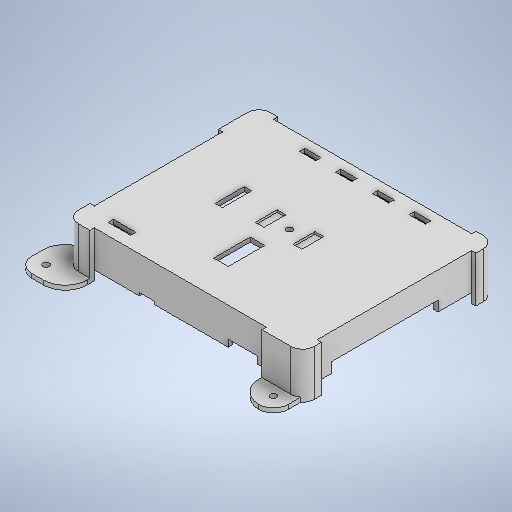
# Autodesk Inventor part: TopCase
Saved by Autodesk Inventor 2025.2 (Build 292293000, 293)
## iProperties
Created: 2026-05-08
Part Number: TopCase
Material: Generic
Document SubType Name: Modeling
Designer: Simon
Density: 1 g/cm^3
Appearance: Default
Author: Simon
Autodesk Inventor part; units mm, degrees
ref_plane "YZ Plane" through (0, 0, 0) normal (1, 0, 0) x (0, 1, 0)
ref_plane "XZ Plane" through (0, 0, 0) normal (0, 1, 0) x (-1, 0, 0)
ref_plane "XY Plane" through (0, 0, 0) normal (0, 0, 1) x (1, 0, 0)
sketch "Sketch1" plane through (0, 0, 0) normal (0, 1, 0) x (-1, 0, 0)
  line L0 (0, 0) -> (-156, 0)
  line L1 (-156, 0) -> (-156, -126)
  line L2 (-156, -126) -> (0, -126)
  line L3 (0, -126) -> (0, 0)
  line L4 (0, 0) -> (-3, 0)
  line L5 (-3, 0) -> (-3, -3)
  line L6 (-3, -3) -> (0, -3)
  line L7 (0, -3) -> (0, 0)
  line L8 (-156, 0) -> (-153, 0)
  line L9 (-153, 0) -> (-153, -3)
  line L10 (-153, -3) -> (-156, -3)
  line L11 (-156, -3) -> (-156, 0)
  line L12 (-156, -126) -> (-153, -126)
  line L13 (-153, -126) -> (-153, -123)
  line L14 (-153, -123) -> (-156, -123)
  line L15 (-156, -123) -> (-156, -126)
  line L16 (0, -126) -> (-3, -126)
  line L17 (-3, -126) -> (-3, -123)
  line L18 (-3, -123) -> (0, -123)
  line L19 (0, -123) -> (0, -126)
  line L20 (-156, 0) -> (-153.2, 0)
  line L21 (-153.2, 0) -> (-153.2, -126)
  line L22 (-153.2, -126) -> (-156, -126)
  line L23 (-156, -126) -> (-156, 0)
  line L24 (0, 0) -> (-2.8, 0)
  line L25 (-2.8, 0) -> (-2.8, -126)
  line L26 (-2.8, -126) -> (0, -126)
  line L27 (0, -126) -> (0, 0)
  line L28 (0, -126) -> (-156, -126)
  line L29 (-156, -126) -> (-156, -123.2)
  line L30 (-156, -123.2) -> (0, -123.2)
  line L31 (0, -123.2) -> (0, -126)
  line L32 (0, 0) -> (-156, 0)
  line L33 (-156, 0) -> (-156, -2.8)
  line L34 (-156, -2.8) -> (0, -2.8)
  line L35 (0, -2.8) -> (0, 0)
  line L36 (-3, -3) -> (-9, -3)
  line L37 (-9, -3) -> (-9, -9)
  line L38 (-9, -9) -> (-3, -9)
  line L39 (-3, -9) -> (-3, -3)
  line L40 (-153, -3) -> (-147, -3)
  line L41 (-147, -3) -> (-147, -9)
  line L42 (-147, -9) -> (-153, -9)
  line L43 (-153, -9) -> (-153, -3)
  line L44 (-153, -123) -> (-147, -123)
  line L45 (-147, -123) -> (-147, -117)
  line L46 (-147, -117) -> (-153, -117)
  line L47 (-153, -117) -> (-153, -123)
  line L48 (-3, -123) -> (-9, -123)
  line L49 (-9, -123) -> (-9, -117)
  line L50 (-9, -117) -> (-3, -117)
  line L51 (-3, -117) -> (-3, -123)
  circle A0 centre (-9, -9) radius 5
  circle A1 centre (-147, -9) radius 5
  circle A2 centre (-147, -117) radius 5
  circle A3 centre (-9, -117) radius 5
  line L52 (0, 0) -> (-44, 0)
  line L53 (-44, 0) -> (-44, -2.8)
  line L54 (-44, -2.8) -> (0, -2.8)
  line L55 (0, -2.8) -> (0, 0)
  line L56 (-156, 0) -> (-54, 0)
  line L57 (-54, 0) -> (-54, -2.8)
  line L58 (-54, -2.8) -> (-156, -2.8)
  line L59 (-156, -2.8) -> (-156, 0)
  line L60 (-156, 0) -> (-153.2, 0)
  line L61 (-153.2, 0) -> (-153.2, -20)
  line L62 (-153.2, -20) -> (-156, -20)
  line L63 (-156, -20) -> (-156, 0)
  line L64 (-156, -126) -> (-153.2, -126)
  line L65 (-153.2, -126) -> (-153.2, -93)
  line L66 (-153.2, -93) -> (-156, -93)
  line L67 (-156, -93) -> (-156, -126)
  line L68 (0, 0) -> (-2.8, 0)
  line L69 (-2.8, 0) -> (-2.8, -14.25)
  line L70 (-2.8, -14.25) -> (0, -14.25)
  line L71 (0, -14.25) -> (0, 0)
  line L72 (0, -126) -> (-2.8, -126)
  line L73 (-2.8, -126) -> (-2.8, -26.25)
  line L74 (-2.8, -26.25) -> (0, -26.25)
  line L75 (0, -26.25) -> (0, -126)
  line L76 (-156, 0) -> (-125, 0)
  line L77 (-125, 0) -> (-125, -2.8)
  line L78 (-125, -2.8) -> (-156, -2.8)
  line L79 (-156, -2.8) -> (-156, 0)
  line L80 (0, 0) -> (-105, 0)
  line L81 (-105, 0) -> (-105, -2.8)
  line L82 (-105, -2.8) -> (0, -2.8)
  line L83 (0, -2.8) -> (0, 0)
  point P0 (0, -26.25)
  point P1 (-2.8, -123.2)
  point P2 (-153.2, -123.2)
  point P3 (-153.2, -2.8)
  point P4 (-2.8, -2.8)
  point P5 (0, -14.25)
  dimension "d0" = 156
  dimension "d1" = 126
  dimension "d5" = 3
  dimension "d6" = 3
  dimension "d7" = 3
  dimension "d8" = 3
  dimension "d9" = 3
  dimension "d10" = 3
  dimension "d11" = 3
  dimension "d12" = 3
  dimension "d13" = 2.8
  dimension "d14" = 2.8
  dimension "d15" = 2.8
  dimension "d16" = 2.8
  dimension "d17" = 6
  dimension "d18" = 6
  dimension "d19" = 6
  dimension "d20" = 6
  dimension "d21" = 6
  dimension "d22" = 6
  dimension "d23" = 6
  dimension "d24" = 6
  dimension "d25" = 10
  dimension "d26" = 10
  dimension "d27" = 10
  dimension "d28" = 10
  dimension "d31" = 44
  dimension "d32" = 102
  dimension "d33" = 20
  dimension "d34" = 33
  dimension "d35" = 14.25
  dimension "d36" = 99.75
  dimension "d53" = 31
  dimension "d54" = 105
  constraints: 168 end point, 42 parallel, 21 horizontal, 21 perpendicular, 11 point on line, 4 centre point, 4 coincident, 1 midpoint
  measures "d0" distance of L2.end L1.end
  measures "d1" distance of L1.end L0.end
  measures "d5" distance of L6.end L5.end
  measures "d6" distance of L5.end L4.end
  measures "d7" distance of L9.end L10.end
  measures "d8" distance of L8.end L9.end
  measures "d9" distance of L14.end L13.end
  measures "d10" distance of L13.end L12.end
  measures "d11" distance of L17.end L18.end
  measures "d12" distance of L16.end L17.end
  measures "d13" distance of L21.end L22.end
  measures "d14" distance of L26.end L25.end
  measures "d15" distance of L28.end L29.end
  measures "d16" distance of L33.end L32.end
  measures "d17" distance of L38.end L37.end
  measures "d18" distance of L37.end L36.end
  measures "d19" distance of L41.end L42.end
  measures "d20" distance of L40.end L41.end
  measures "d21" distance of L46.end L45.end
  measures "d22" distance of L45.end L44.end
  measures "d23" distance of L49.end L50.end
  measures "d24" distance of L48.end L49.end
  measures "d25" diameter of A0
  measures "d26" diameter of A1
  measures "d27" diameter of A2
  measures "d28" diameter of A3
  measures "d31" distance of L54.end L53.end
  measures "d32" distance of L57.end L58.end
  measures "d33" distance of L60.end L61.end
  measures "d34" distance of L65.end L64.end
  measures "d35" distance of L69.end L68.end
  measures "d36" distance of L72.end L73.end
  measures "d53" distance of L77.end L78.end
  measures "d54" distance of L82.end L81.end
extrude "Extrusion1" add sketch "Sketch1" along normal blind 3 contours L3 L34 L25 L0 | L25 L34 L5 L0 | L3 L6 L25 L34 | L5 L34 L53 L0 | L25 L6 L5 L34 | L3 L70 L25 L6 | L53 L34 L57 L0 | L40 L41 A1 L42 L43 | L47 L46 A2 L45 L44 | L48 L49 A3 L50 L51 | L39 L38 A0 L37 L36 | L5 L6 L25 L18 L17 L30 L13 L14 L21 L10 L9 L34 | L3 L74 L25 L70 | L57 L34 L81 L0 | L3 L18 L25 L74 | L81 L34 L77 L0 | L3 L30 L25 L18 | L77 L34 L9 L0 | A0 L38 L37 | L37 L38 A0 | L25 L30 L17 L18 | L3 L2 L25 L30 | L9 L34 L21 L0 | L25 L2 L17 L30 | L21 L34 L1 L0 | L9 L10 L21 L34 | L17 L2 L13 L30 | L21 L10 L1 L34 | L30 L21 L14 L13 | L13 L2 L21 L30 | A3 L50 L49 | L49 L50 A3 | L21 L62 L1 L10 | L30 L1 L14 L21 | L21 L2 L1 L30 | L21 L66 L1 L62 | A1 L42 L41 | L41 L42 A1 | L14 L1 L66 L21 | A2 L46 L45 | L45 L46 A2
fillet "Fillet1" radius 5 4 edges at (156, 1.5, 0) (156, 1.5, -126) (0, 1.5, 0) (0, 1.5, -126)
extrude "Extrusion2" add sketch "Sketch1" against normal blind 21.8 contours A0 L38 L37 | L37 L38 A0 | A3 L50 L49 | L49 L50 A3 | A1 L42 L41 | L41 L42 A1 | A2 L46 L45 | L45 L46 A2
extrude "Extrusion3" add sketch "Sketch1" against normal blind 22 contours L3 L34 L25 L0 | L25 L34 L5 L0 | L3 L6 L25 L34 | L5 L34 L53 L0 | L3 L70 L25 L6 | L57 L34 L81 L0 | L3 L18 L25 L74 | L3 L30 L25 L18 | L77 L34 L9 L0 | L3 L2 L25 L30 | L9 L34 L21 L0 | L25 L2 L17 L30 | L21 L34 L1 L0 | L17 L2 L13 L30 | L21 L10 L1 L34 | L13 L2 L21 L30 | L21 L62 L1 L10 | L30 L1 L14 L21 | L21 L2 L1 L30 | L14 L1 L66 L21
fillet "Fillet2" radius 5 4 edges at (0, -11, 0) (156, -11, 0) (156, -11, -126) (0, -11, -126)
fillet "Fillet3" radius 5 4 edges at (2.8, -11, -2.8) (2.8, -11, -123.2) (153.2, -11, -2.8) (153.2, -11, -123.2)
sketch "Sketch2" plane through (9, -21.8, -9) normal (0, -1, 0) x (1, 0, 0)
  circle A0 centre (0, 0) radius 2.15
  circle A1 centre (138, 0) radius 5 projected
  circle A2 centre (138, 0) radius 2.15
  circle A3 centre (138, -108) radius 5 projected
  circle A4 centre (138, -108) radius 2.15
  circle A5 centre (0, -108) radius 5 projected
  circle A6 centre (0, -108) radius 2.15
  point P0 (-9, 9)
  dimension "d41" = 4.3
  dimension "d42" = 4.3
  dimension "d43" = 4.3
  dimension "d44" = 4.3
  constraints: 4 centre point, 3 coincident
  measures "d41" diameter of A0
  measures "d42" diameter of A2
  measures "d43" diameter of A4
  measures "d44" diameter of A6
extrude "Extrusion4" cut sketch "Sketch2" against normal blind 8 contours A0 | A2 | A4 | A6
extrude "Extrusion5" add sketch "Sketch1" against normal blind 20 contours L53 L34 L57 L0
extrude "Extrusion6" add sketch "Sketch1" against normal blind 15 contours L21 L66 L1 L62
extrude "Extrusion7" add sketch "Sketch1" against normal blind 17 contours L3 L74 L25 L70
extrude "Extrusion8" add sketch "Sketch1" against normal blind 20 contours L81 L34 L77 L0
chamfer "Chamfer1" distance 2.8 angle 45 1 edges at (115, -20, 0)
sketch "Sketch3" plane through (0, 3, 0) normal (0, 1, 0) x (1, 0, 0)
  arc A0 (0, 5) -> (5, 0) centre (5, 5) ccw projected
  line L0 (0, 0) -> (5, 0)
  line L1 (5, 0) -> (5, 5)
  line L2 (5, 5) -> (0, 5)
  line L3 (0, 5) -> (0, 0)
  arc A1 (151, 0) -> (156, 5) centre (151, 5) ccw projected
  line L4 (151, 5) -> (156, 5)
  line L5 (156, 5) -> (156, 0)
  line L6 (156, 0) -> (151, 0)
  line L7 (151, 0) -> (151, 5)
  arc A2 (156, 121) -> (151, 126) centre (151, 121) ccw projected
  line L8 (151, 121) -> (156, 121)
  line L9 (156, 121) -> (156, 126)
  line L10 (156, 126) -> (151, 126)
  line L11 (151, 126) -> (151, 121)
  arc A3 (5, 126) -> (0, 121) centre (5, 121) ccw projected
  line L12 (5, 121) -> (0, 121)
  line L13 (0, 121) -> (0, 126)
  line L14 (0, 126) -> (5, 126)
  line L15 (5, 126) -> (5, 121)
  line L16 (0, 0) -> (10, 0)
  line L17 (10, 0) -> (10, 10)
  line L18 (10, 10) -> (0, 10)
  line L19 (0, 10) -> (0, 0)
  line L20 (10, 10) -> (-3, 10)
  line L21 (-3, 10) -> (-3, -3)
  line L22 (-3, -3) -> (10, -3)
  line L23 (10, -3) -> (10, 10)
  line L24 (156, 0) -> (146, 0)
  line L25 (146, 0) -> (146, 10)
  line L26 (146, 10) -> (156, 10)
  line L27 (156, 10) -> (156, 0)
  line L28 (156, 126) -> (146, 126)
  line L29 (146, 126) -> (146, 116)
  line L30 (146, 116) -> (156, 116)
  line L31 (156, 116) -> (156, 126)
  line L32 (0, 126) -> (10, 126)
  line L33 (10, 126) -> (10, 116)
  line L34 (10, 116) -> (0, 116)
  line L35 (0, 116) -> (0, 126)
  line L36 (10, 116) -> (-3, 116)
  line L37 (-3, 116) -> (-3, 129)
  line L38 (-3, 129) -> (10, 129)
  line L39 (10, 129) -> (10, 116)
  line L40 (146, 116) -> (159, 116)
  line L41 (159, 116) -> (159, 129)
  line L42 (159, 129) -> (146, 129)
  line L43 (146, 129) -> (146, 116)
  line L44 (146, 10) -> (159, 10)
  line L45 (159, 10) -> (159, -3)
  line L46 (159, -3) -> (146, -3)
  line L47 (146, -3) -> (146, 10)
  arc A4 (0, 5) -> (5, 0) centre (5, 5) ccw
  arc A5 (-3, 5) -> (5, -3) centre (5, 5) ccw
  arc A6 (5, 129) -> (-3, 121) centre (5, 121) ccw
  arc A7 (159, 121) -> (151, 129) centre (151, 121) ccw
  line L48 (151, 126) -> (5, 126) projected
  arc A8 (156, 121) -> (151, 126) centre (151, 121) ccw
  arc A9 (151, -3) -> (159, 5) centre (151, 5) ccw
  arc A10 (151, 0) -> (156, 5) centre (151, 5) ccw
  arc A11 (5, 126) -> (0, 121) centre (5, 121) ccw
  arc A12 (0, 5) -> (5, 0) centre (5, 5) ccw
  line L49 (-3, 10) -> (0, 10)
  line L50 (0, 10) -> (0, 12.5587)
  line L51 (5, 0) -> (151, 0) projected
  line L52 (10, -3) -> (13, -3)
  line L53 (13, -3) -> (13, 0)
  line L54 (13, 0) -> (10, 0)
  line L55 (10, 0) -> (10, -3)
  line L56 (-3, 10) -> (0, 10)
  line L57 (0, 10) -> (0, 13)
  line L58 (0, 13) -> (-3, 13)
  line L59 (-3, 13) -> (-3, 10)
  line L60 (146, -3) -> (131, -3)
  line L61 (131, -3) -> (131, 0)
  line L62 (131, 0) -> (146, 0)
  line L63 (146, 0) -> (146, -3)
  line L64 (0, 26.25) -> (0, 121) projected
  line L65 (-3, 116) -> (0, 116)
  line L66 (0, 116) -> (0, 101)
  line L67 (0, 101) -> (-3, 101)
  line L68 (-3, 101) -> (-3, 116)
  point P0 (151, 0)
  point P1 (5, 0)
  point P2 (0, 5)
  point P3 (0, 121)
  dimension "d60" = 10
  dimension "d61" = 10
  dimension "d62" = 13
  dimension "d63" = 13
  dimension "d64" = 10
  dimension "d65" = 10
  dimension "d66" = 10
  dimension "d67" = 10
  dimension "d68" = 10
  dimension "d69" = 10
  dimension "d70" = 13
  dimension "d71" = 13
  dimension "d72" = 13
  dimension "d73" = 13
  dimension "d74" = 13
  dimension "d75" = 13
  dimension "d76" = 3
  dimension "d77" = 3
  dimension "d78" = 15
  dimension "d79" = 15
  constraints: 132 end point, 32 parallel, 20 point on line, 19 point on circle, 17 horizontal, 17 perpendicular, 9 centre point, 9 coincident, 1 midpoint
  measures "d60" distance of L18.end L17.end
  measures "d61" distance of L17.end L16.end
  measures "d62" distance of L22.end L21.end
  measures "d63" distance of L21.end L20.end
  measures "d64" distance of L25.end L26.end
  measures "d65" distance of L24.end L25.end
  measures "d66" distance of L30.end L29.end
  measures "d67" distance of L29.end L28.end
  measures "d68" distance of L33.end L34.end
  measures "d69" distance of L32.end L33.end
  measures "d70" distance of L37.end L38.end
  measures "d71" distance of L36.end L37.end
  measures "d72" distance of L42.end L41.end
  measures "d73" distance of L41.end L40.end
  measures "d74" distance of L45.end L46.end
  measures "d75" distance of L44.end L45.end
  measures "d76" distance of L54.end L53.end
  measures "d77" distance of L57.end L56.end
  measures "d78" distance of L61.end L62.end
  measures "d79" distance of L65.end L66.end
extrude "Extrusion9" add sketch "Sketch3" against normal blind 31.5 contours A0 L0 L3 | L3 L0 L16 L23 L22 A5 L21 L20 L19 | L20 L59 L58 L57 L50 | L51 L53 L52 L23 | A1 L5 L6 | L6 L5 L27 L44 L45 A9 L46 L47 L24 | L47 L60 L61 L51 | A2 L10 L9 | L9 L10 L28 L43 L42 A7 L41 L40 L31 | A3 L13 L14 | L14 L13 L35 L36 L37 A6 L38 L39 L32 | L64 L67 L68 L36
sketch "Sketch4" plane through (0, -28.5, 0) normal (0, -1, 0) x (1, 0, 0)
  line L0 (0, 0) -> (156, 0)
  line L1 (156, 0) -> (156, -126)
  line L2 (156, -126) -> (0, -126)
  line L3 (0, -126) -> (0, 0)
  arc A0 (156, -5) -> (151, 0) centre (151, -5) ccw projected
  line L4 (156, -5) -> (156, 0)
  line L5 (156, 0) -> (151, 0)
  line L6 (156, 0) -> (151, 0)
  line L7 (151, 0) -> (151, -5)
  line L8 (151, -5) -> (156, -5)
  line L9 (156, -5) -> (156, 0)
  circle A1 centre (151, -5) radius 5
  line L10 (156, 0) -> (131, 0)
  line L11 (131, 0) -> (131, 20)
  line L12 (131, 20) -> (156, 20)
  line L13 (156, 20) -> (156, 0)
  arc A2 (5, 0) -> (0, -5) centre (5, -5) ccw projected
  line L14 (0, 0) -> (5, 0)
  line L15 (5, 0) -> (5, -5)
  line L16 (5, -5) -> (0, -5)
  line L17 (0, -5) -> (0, 0)
  arc A3 (5, 0) -> (0, -5) centre (5, -5) ccw
  line L18 (-3, 3) -> (0, 3)
  line L19 (0, 3) -> (0, -13)
  line L20 (0, -13) -> (-3, -13)
  line L21 (-3, -13) -> (-3, 3)
  line L22 (-3, 3) -> (13, 3)
  line L23 (13, 3) -> (13, 0)
  line L24 (13, 0) -> (-3, 0)
  line L25 (-3, 0) -> (-3, 3)
  line L26 (-3, 3) -> (-23, 3)
  line L27 (-23, 3) -> (-23, 20)
  line L28 (-23, 20) -> (-3, 20)
  line L29 (-3, 20) -> (-3, 3)
  line L30 (-23, 20) -> (13, 20)
  line L31 (13, 20) -> (13, -13)
  line L32 (13, -13) -> (-23, -13)
  line L33 (-23, -13) -> (-23, 20)
  arc A4 (0, -121) -> (5, -126) centre (5, -121) ccw projected
  line L34 (5, -121) -> (0, -121)
  line L35 (0, -121) -> (0, -126)
  line L36 (0, -126) -> (5, -126)
  line L37 (5, -126) -> (5, -121)
  circle A5 centre (5, -121) radius 5
  line L38 (-3, -129) -> (10, -129)
  line L39 (10, -129) -> (10, -101)
  line L40 (10, -101) -> (-3, -101)
  line L41 (-3, -101) -> (-3, -129)
  line L42 (-3, -129) -> (-23, -129)
  line L43 (-23, -129) -> (-23, -146)
  line L44 (-23, -146) -> (-3, -146)
  line L45 (-3, -146) -> (-3, -129)
  line L46 (-23, -146) -> (10, -146)
  line L47 (10, -146) -> (10, -101)
  line L48 (10, -101) -> (-23, -101)
  line L49 (-23, -101) -> (-23, -146)
  line L50 (-3, -129) -> (156, -129)
  line L51 (156, -129) -> (156, 0)
  line L52 (156, 0) -> (-3, 0)
  line L53 (-3, 0) -> (-3, -129)
  line L54 (-3, -129) -> (159, -129)
  line L55 (159, -129) -> (159, 6)
  line L56 (159, 6) -> (-3, 6)
  line L57 (-3, 6) -> (-3, -129)
  line L58 (-3, -146) -> (-20, -146)
  line L59 (-20, -146) -> (-20, 20)
  line L60 (-20, 20) -> (-3, 20)
  line L61 (-3, 20) -> (-3, -146)
  line L62 (10, -101) -> (-20, -101)
  line L63 (-20, -101) -> (-20, -126)
  line L64 (-20, -126) -> (10, -126)
  line L65 (10, -126) -> (10, -101)
  point P0 (0, -101)
  point P1 (-20, -13)
  dimension "d82" = 156
  dimension "d83" = 126
  dimension "d84" = 25
  dimension "d85" = 20
  dimension "d86" = 16
  dimension "d87" = 16
  dimension "d88" = 20
  dimension "d89" = 17
  dimension "d90" = 28
  dimension "d91" = 20
  dimension "d92" = 17
  dimension "d95" = 17
  constraints: 132 end point, 32 parallel, 16 horizontal, 16 perpendicular, 6 point on line, 3 coincident, 2 point on circle, 1 centre point, 1 horizontal alignment, 1 vertical alignment, 4 other
  measures "d82" distance of L1.end L2.end
  measures "d83" distance of L0.end L1.end
  measures "d84" distance of L11.end L12.end
  measures "d85" distance of L10.end L11.end
  measures "d86" distance of L18.end L19.end
  measures "d87" distance of L23.end L24.end
  measures "d88" distance of L27.end L28.end
  measures "d89" distance of L26.end L27.end
  measures "d90" distance of L39.end L38.end
  measures "d91" distance of L44.end L43.end
  measures "d92" distance of L43.end L42.end
  measures "d95" distance of L59.end L60.end
extrude "Extrusion10" add sketch "Sketch4" against normal blind 3 contours L19 L22 L23 L0 | L0 A2 L3 | L24 L21 L18 L19 | L3 L20 L21 L24 | L18 L29 L56 L31 L22 | L21 L32 L59 L26 | L26 L59 L28 L29 | L11 L56 L13 L0 | L3 L64 L41 L40 | L29 L30 L31 L56 | L41 L64 L59 L48 | L0 L1 A0 | L11 L12 L13 L56 | A4 L2 L3
fillet "Fillet4" radius 10 3 edges at (156, -27, 20) (-20, -27, 20) (-20, -27, -126)
sketch "Sketch5" plane through (0, -25.5, 0) normal (0, 1, 0) x (1, 0, 0)
  arc A0 (-20, -10) -> (-10, -20) centre (-10, -10) ccw projected
  line L0 (-20, -20) -> (-10, -20)
  line L1 (-10, -20) -> (-10, -10)
  line L2 (-10, -10) -> (-20, -10)
  line L3 (-20, -10) -> (-20, -20)
  arc A1 (-10, 126) -> (-20, 116) centre (-10, 116) ccw projected
  line L4 (-20, 126) -> (-10, 126)
  line L5 (-10, 126) -> (-10, 116)
  line L6 (-10, 116) -> (-20, 116)
  line L7 (-20, 116) -> (-20, 126)
  arc A2 (146, -20) -> (156, -10) centre (146, -10) ccw projected
  line L8 (156, -20) -> (146, -20)
  line L9 (146, -20) -> (146, -10)
  line L10 (146, -10) -> (156, -10)
  line L11 (156, -10) -> (156, -20)
  circle A3 centre (-10, 116) radius 2.15
  circle A4 centre (-10, -10) radius 2.15
  circle A5 centre (146, -10) radius 2.15
  point P0 (0, 0)
  dimension "d97" = 4.3
  dimension "d98" = 4.3
  dimension "d99" = 4.3
  constraints: 24 end point, 6 parallel, 3 centre point, 3 coincident, 3 horizontal, 3 perpendicular, 2 point on line
  measures "d97" diameter of A3
  measures "d98" diameter of A4
  measures "d99" diameter of A5
extrude "Extrusion11" cut sketch "Sketch5" against normal blind 3 contours A4 L1 L2 | L2 L1 A4 | A3 L6 L5 | L5 L6 A3 | A5 L10 L9 | L9 L10 A5
fillet "Fillet5" radius 15 4 edges at (13, -27, 20) (131, -27, 20) (-20, -27, -101) (-20, -27, -13)
sketch "Sketch6" plane through (0, 3, 0) normal (0, 1, 0) x (1, 0, 0)
  line L0 (0, 0) -> (14.5, 0)
  line L1 (14.5, 0) -> (14.5, 8)
  line L2 (14.5, 8) -> (0, 8)
  line L3 (0, 8) -> (0, 0)
  line L4 (14.5, 8) -> (30, 8)
  line L5 (30, 8) -> (30, 11.6)
  line L6 (30, 11.6) -> (14.5, 11.6)
  line L7 (14.5, 11.6) -> (14.5, 8)
  line L8 (156, 0) -> (82, 0)
  line L9 (82, 0) -> (82, 23)
  line L10 (82, 23) -> (156, 23)
  line L11 (156, 23) -> (156, 0)
  line L12 (82, 23) -> (72, 23)
  line L13 (72, 23) -> (72, 48)
  line L14 (72, 48) -> (82, 48)
  line L15 (82, 48) -> (82, 23)
  line L16 (156, 10) -> (156, 116) projected
  line L17 (10, 126) -> (146, 126) projected
  line L18 (156, 116) -> (146, 116)
  line L19 (146, 116) -> (146, 126)
  line L20 (146, 126) -> (156, 126)
  line L21 (156, 126) -> (156, 116)
  line L22 (0, 126) -> (40, 126)
  line L23 (40, 126) -> (40, 76)
  line L24 (40, 76) -> (0, 76)
  line L25 (0, 76) -> (0, 126)
  line L26 (40, 76) -> (45, 76)
  line L27 (45, 76) -> (45, 56)
  line L28 (45, 56) -> (40, 56)
  line L29 (40, 56) -> (40, 76)
  line L30 (156, 126) -> (124.4, 126)
  line L31 (124.4, 126) -> (124.4, 119.5)
  line L32 (124.4, 119.5) -> (156, 119.5)
  line L33 (156, 119.5) -> (156, 126)
  line L34 (124.4, 119.5) -> (113.3, 119.5)
  line L35 (113.3, 119.5) -> (113.3, 115.9)
  line L36 (113.3, 115.9) -> (124.4, 115.9)
  line L37 (124.4, 115.9) -> (124.4, 119.5)
  line L38 (113.3, 119.5) -> (99.25, 119.5)
  line L39 (99.25, 119.5) -> (88.15, 119.5)
  line L40 (88.15, 119.5) -> (73.85, 119.5)
  line L41 (73.85, 119.5) -> (62.75, 119.5)
  line L42 (62.75, 119.5) -> (49.05, 119.5)
  line L43 (62.75, 119.5) -> (77, 119.5)
  line L44 (88.15, 119.5) -> (102, 119.5)
  line L45 (62.75, 119.5) -> (73.85, 119.5)
  line L46 (73.85, 119.5) -> (73.85, 115.9)
  line L47 (73.85, 115.9) -> (62.75, 115.9)
  line L48 (62.75, 115.9) -> (62.75, 119.5)
  line L49 (88.15, 119.5) -> (99.25, 119.5)
  line L50 (99.25, 119.5) -> (99.25, 115.9)
  line L51 (99.25, 115.9) -> (88.15, 115.9)
  line L52 (88.15, 115.9) -> (88.15, 119.5)
  line L53 (49.05, 119.5) -> (37.95, 119.5)
  line L54 (37.95, 119.5) -> (37.95, 115.9)
  line L55 (37.95, 115.9) -> (49.05, 115.9)
  line L56 (49.05, 115.9) -> (49.05, 119.5)
  line L57 (0, 101) -> (0, 13) projected
  line L58 (13, 0) -> (131, 0) projected
  line L59 (156, 126) -> (81, 126)
  line L60 (81, 126) -> (81, 66)
  line L61 (81, 66) -> (156, 66)
  line L62 (156, 66) -> (156, 126)
  circle A0 centre (81, 66) radius 2.15
  point P0 (99.25, 117.7)
  point P1 (88.15, 117.7)
  dimension "d103" = 14.5
  dimension "d104" = 8
  dimension "d105" = 15.5
  dimension "d106" = 3.6
  dimension "d107" = 74
  dimension "d108" = 23
  dimension "d109" = 10
  dimension "d110" = 25
  dimension "d111" = 40
  dimension "d112" = 50
  dimension "d113" = 5
  dimension "d114" = 20
  dimension "d115" = 31.6
  dimension "d116" = 6.5
  dimension "d117" = 11.1
  dimension "d118" = 3.6
  dimension "d119" = 14.05
  dimension "d120" = 11.1
  dimension "d121" = 14.3
  dimension "d122" = 11.1
  dimension "d123" = 13.7
  dimension "d130" = 3.6
  dimension "d131" = 11.1
  dimension "d132" = 3.6
  dimension "d133" = 11.1
  dimension "d134" = 11.1
  dimension "d135" = 0
  dimension "d136" = 0
  dimension "d137" = 0
  dimension "d138" = 75
  dimension "d139" = 60
  dimension "d140" = 4.3
  constraints: 118 end point, 26 parallel, 16 horizontal, 13 perpendicular, 6 point on line, 2 midpoint, 1 centre point, 1 coincident
  measures "d103" distance of L2.end L1.end
  measures "d104" distance of L1.end L0.end
  measures "d105" distance of L6.end L5.end
  measures "d106" distance of L5.end L4.end
  measures "d107" distance of L9.end L10.end
  measures "d108" distance of L8.end L9.end
  measures "d109" distance of L13.end L14.end
  measures "d110" distance of L12.end L13.end
  measures "d111" distance of L23.end L24.end
  measures "d112" distance of L22.end L23.end
  measures "d113" distance of L27.end L28.end
  measures "d114" distance of L26.end L27.end
  measures "d115" distance of L32.end L31.end
  measures "d116" distance of L31.end L30.end
  measures "d117" distance of L36.end L35.end
  measures "d118" distance of L35.end L34.end
  measures "d119" distance of L34.end L38.end
  measures "d120" distance of L38.end L39.end
  measures "d121" distance of L39.end L40.end
  measures "d122" distance of L40.end L41.end
  measures "d123" distance of L41.end L42.end
  measures "d130" distance between parallel lines of L51 L49
  measures "d131" distance of L55.end L54.end
  measures "d132" distance of L54.end L53.end
  measures "d133" distance of point (99.25, 117.7) point (88.15, 117.7)
  measures "d134" distance between parallel lines of L46 L48
  measures "d135" distance between parallel lines of L25 L57
  measures "d136" distance between parallel lines of L16 L11
  measures "d137" distance between parallel lines of L58 L8
  measures "d138" distance of L61.end L60.end
  measures "d139" distance of L60.end L59.end
  measures "d140" diameter of A0
extrude "Extrusion13" cut sketch "Sketch6" against normal through all contours L7 L6 L5 L4 | L12 L13 L14 L15 | L26 L27 L28 L29 | A0 L60 L61 | L61 L60 A0 | L37 L36 L35 L34 | L39 L50 L51 L52 | L46 L47 L48 L41 | L53 L56 L55 L23 | L23 L55 L54 L53
sketch "Sketch7" plane through (0, 3, 0) normal (0, 1, 0) x (1, 0, 0)
  circle A0 centre (81, 66) radius 2.15 projected
  circle A1 centre (81, 66) radius 2.15
  line L0 (71, 73.5) -> (91, 73.5)
  line L1 (91, 73.5) -> (91, 58.5)
  line L2 (91, 58.5) -> (71, 58.5)
  line L3 (71, 58.5) -> (71, 73.5)
  line L4 (71, 73.5) -> (91, 58.5) construction
  line L5 (91, 73.5) -> (71, 58.5) construction
  line L6 (65, 58.5) -> (97, 58.5)
  line L7 (97, 58.5) -> (97, 73.5)
  line L8 (97, 73.5) -> (65, 73.5)
  line L9 (65, 73.5) -> (65, 58.5)
  line L10 (65, 58.5) -> (97, 73.5) construction
  line L11 (97, 58.5) -> (65, 73.5) construction
  point P0 (0, 0)
  dimension "d141" = 20
  dimension "d142" = 15
  dimension "d143" = 32
  constraints: 24 end point, 4 midpoint, 4 parallel, 2 horizontal, 2 perpendicular, 1 centre point, 1 coincident, 1 point on line
  measures "d141" distance of L1.end L2.end
  measures "d142" distance of L0.end L1.end
  measures "d143" distance of L8.end L7.end
extrude "Extrusion14" cut sketch "Sketch7" against normal blind 1.5 contours L3 L6 L9 L8 | L8 L7 L6 L1
body "Solid1"
